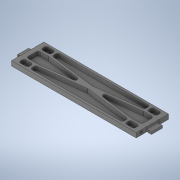
# Autodesk Inventor part: Cockpit_battery_front_frame
Saved by Autodesk Inventor 2020.4 (Build 244396000, 396)
## iProperties
Created: 2022-01-28
Part Number: Cockpit_battery_front_frame
Material: アセタール樹脂、黒
Document SubType Name: Modeling
Designer: Masato Kubotera
Density: 1.425 g/cm^3
Appearance: 滑らか - 黒
Description: POM T5
Author: Masato Kubotera
Autodesk Inventor part; units mm, degrees
ref_plane "XZ Plane" through (0, 0, 0) normal (0, 1, 0) x (-1, 0, 0)
ref_plane "XY Plane" through (0, 0, 0) normal (0, 0, 1) x (1, 0, 0)
derived "Cockpit_side_frame.ipt"
sketch "スケッチ2" plane through (0, 0, 0) normal (0, 1, 0) x (-1, 0, 0)
  line L0 (-28.5, -22.5) -> (86.5, -22.5) construction
  line L1 (86.5, -22.5) -> (86.5, -138.5)
  line L2 (86.5, -96) -> (-28.5, -96) construction
  line L3 (-28.5, -96) -> (-28.5, -22.5) construction
  line L4 (-28.5, -22.5) -> (86.5, -96) construction
  line L5 (86.5, -22.5) -> (-28.5, -96) construction
  line L6 (36.5, -101) -> (36.5, -133.5)
  line L7 (41.5, -138.5) -> (86.5, -138.5)
  arc A0 (62.6349, -67.15) -> (61.15, -68.6349) centre (61.8925, -67.8925) ccw
  arc A1 (71.15, -69.2849) -> (69.6651, -67.8) centre (70.4075, -68.5425) ccw
  line L8 (63.3349, -67.8) -> (69.6651, -67.8)
  line L9 (62.6349, -67.15) -> (70.3651, -67.15)
  line L10 (61.9, -67.85) -> (71.1, -67.85) construction
  arc A2 (63.3349, -67.8) -> (61.85, -69.2849) centre (62.5925, -68.5425) ccw
  line L11 (61.2, -67.2) -> (71.8, -67.2) construction
  line L12 (71.15, -69.2849) -> (71.15, -80.2151)
  line L13 (71.8, -74.75) -> (61.2, -74.75) construction
  line L14 (71.85, -68.6349) -> (71.85, -80.8651)
  line L15 (71.1, -67.85) -> (71.1, -81.65) construction
  line L16 (61.85, -69.2849) -> (61.85, -80.2151)
  line L17 (71.8, -67.2) -> (71.8, -82.3) construction
  line L18 (61.15, -68.6349) -> (61.15, -80.8651)
  line L19 (66.5, -67.2) -> (66.5, -82.3) construction
  line L20 (61.9, -81.65) -> (61.9, -67.85) construction
  line L21 (71.1, -67.85) -> (61.9, -81.65) construction
  line L22 (71.8, -67.2) -> (61.2, -82.3) construction
  line L23 (61.2, -67.2) -> (71.8, -82.3) construction
  line L24 (61.2, -82.3) -> (61.2, -67.2) construction
  line L25 (61.9, -67.85) -> (71.1, -81.65) construction
  arc A3 (71.85, -68.6349) -> (70.3651, -67.15) centre (71.1075, -67.8925) ccw
  line L26 (71.1, -81.65) -> (61.9, -81.65) construction
  line L27 (71.8, -82.3) -> (61.2, -82.3) construction
  arc A4 (61.85, -80.2151) -> (63.3349, -81.7) centre (62.5925, -80.9575) ccw
  arc A5 (61.15, -80.8651) -> (62.6349, -82.35) centre (61.8925, -81.6075) ccw
  line L28 (63.3349, -81.7) -> (69.6651, -81.7)
  line L29 (62.6349, -82.35) -> (70.3651, -82.35)
  arc A6 (69.6651, -81.7) -> (71.15, -80.2151) centre (70.4075, -80.9575) ccw
  arc A7 (70.3651, -82.35) -> (71.85, -80.8651) centre (71.1075, -81.6075) ccw
  line L30 (-23.5, -22.5) -> (-28.5, -27.5)
  line L31 (-28.5, -59.25) -> (86.5, -59.25) construction
  line L32 (29, -22.5) -> (29, -96) construction
  line L33 (-23.5, -96) -> (-28.5, -91)
  line L34 (-28.5, -27.5) -> (-28.5, -91)
  line L35 (-21, -25) -> (-26, -25) construction
  line L36 (-26, -25) -> (-26, -93.5) construction
  line L37 (-26, -93.5) -> (-21, -93.5) construction
  line L38 (-21, -93.5) -> (-21, -25) construction
  line L39 (-21, -25) -> (-26, -93.5) construction
  line L40 (-26, -25) -> (-21, -93.5) construction
  line L41 (-26.05, -46.7) -> (-20.95, -46.7)
  line L42 (-20.95, -46.7) -> (-20.95, -71.8)
  line L43 (-20.95, -71.8) -> (-26.05, -71.8)
  line L44 (-26.05, -71.8) -> (-26.05, -46.7)
  line L45 (-26.05, -46.7) -> (-20.95, -71.8) construction
  line L46 (-20.95, -46.7) -> (-26.05, -71.8) construction
  line L47 (-26, -46.75) -> (-21, -46.75) construction
  line L48 (-26, -71.75) -> (-21, -71.75) construction
  line L49 (-23.5, -25) -> (-23.5, -93.5) construction
  circle A8 centre (-23.5, -35) radius 3
  circle A9 centre (-23.5, -35) radius 1.6
  arc A10 (-24.5651, -46.7) -> (-26.05, -48.1849) centre (-25.3075, -47.4425) ccw
  arc A11 (-20.95, -48.1849) -> (-22.4349, -46.7) centre (-21.6925, -47.4425) ccw
  arc A12 (-22.4349, -71.8) -> (-20.95, -70.3151) centre (-21.6925, -71.0575) ccw
  arc A13 (-26.05, -70.3151) -> (-24.5651, -71.8) centre (-25.3075, -71.0575) ccw
  circle A14 centre (-23.5, -83.5) radius 1.6
  circle A15 centre (-23.5, -83.5) radius 3
  line L50 (31.5, -96) -> (36.5, -101)
  line L51 (-23.5, -96) -> (31.5, -96)
  line L52 (79, -61) -> (-21, -61) construction
  line L53 (-21, -61) -> (-21, -56) construction
  line L54 (-21, -56) -> (79, -56) construction
  line L55 (79, -56) -> (79, -61) construction
  line L56 (79, -61) -> (-21, -56) construction
  line L57 (-21, -61) -> (79, -56) construction
  line L58 (-21, -58.5) -> (79, -58.5) construction
  line L59 (29, -56) -> (29, -61) construction
  line L60 (4, -56) -> (4, -61) construction
  line L61 (54.05, -55.95) -> (3.95, -55.95)
  line L62 (3.95, -55.95) -> (3.95, -61.05)
  line L63 (3.95, -61.05) -> (54.05, -61.05)
  line L64 (54.05, -61.05) -> (54.05, -55.95)
  line L65 (54.05, -55.95) -> (3.95, -61.05) construction
  line L66 (3.95, -55.95) -> (54.05, -61.05) construction
  arc A16 (5.4349, -55.95) -> (3.95, -57.4349) centre (4.6925, -56.6925) ccw
  circle A17 centre (-3.5, -58.5) radius 3
  circle A18 centre (-3.5, -58.5) radius 1.6
  line L67 (54, -56) -> (54, -61) construction
  arc A19 (54.05, -57.4349) -> (52.5651, -55.95) centre (53.3075, -56.6925) ccw
  circle A20 centre (61.5, -58.5) radius 3
  circle A21 centre (61.5, -58.5) radius 1.6
  arc A22 (3.95, -59.5651) -> (5.4349, -61.05) centre (4.6925, -60.3075) ccw
  arc A23 (52.5651, -61.05) -> (54.05, -59.5651) centre (53.3075, -60.3075) ccw
  line L68 (-21, -88.5) -> (79, -88.5) construction
  line L69 (79, -88.5) -> (79, -93.5) construction
  line L70 (79, -93.5) -> (-21, -93.5) construction
  line L71 (-21, -93.5) -> (-21, -88.5) construction
  line L72 (-21, -88.5) -> (79, -93.5) construction
  line L73 (79, -88.5) -> (-21, -93.5) construction
  line L74 (-21, -91) -> (79, -91) construction
  line L75 (29, -88.5) -> (29, -93.5) construction
  line L76 (54.05, -91.05) -> (3.95, -91.05)
  line L77 (3.95, -91.05) -> (3.95, -88.45)
  line L78 (3.95, -88.45) -> (54.05, -88.45)
  line L79 (54.05, -88.45) -> (54.05, -91.05)
  line L80 (54.05, -91.05) -> (3.95, -88.45) construction
  line L81 (3.95, -91.05) -> (54.05, -88.45) construction
  line L82 (4, -88.5) -> (4, -91) construction
  line L83 (54, -88.5) -> (54, -91) construction
  line L84 (4, -89.75) -> (54, -89.75) construction
  arc A24 (6.05, -88.45) -> (3.95, -88.45) centre (5, -88.45) ccw
  arc A25 (54.05, -88.45) -> (51.95, -88.45) centre (53, -88.45) ccw
  arc A26 (51.95, -91.05) -> (54.05, -91.05) centre (53, -91.05) ccw
  arc A27 (3.95, -91.05) -> (6.05, -91.05) centre (5, -91.05) ccw
  circle A28 centre (-3.5, -91) radius 3
  circle A29 centre (-3.5, -91) radius 1.6
  circle A30 centre (61.5, -91) radius 3 construction
  circle A31 centre (61.5, -91) radius 1.6 construction
  line L85 (-23.5, -22.5) -> (64.25, -22.5)
  line L86 (64.25, -22.5) -> (64.25, -17.5)
  line L87 (64.25, -17.5) -> (72.25, -17.5)
  line L88 (72.25, -17.5) -> (72.25, -22.5)
  line L89 (72.25, -22.5) -> (79, -22.5)
  line L90 (79, -22.5) -> (79, -17.5)
  line L91 (86.5, -22.5) -> (86.5, -20)
  line L92 (79, -17.5) -> (84, -17.5)
  line L93 (84, -17.5) -> (86.5, -20)
  line L94 (68.25, -17.5) -> (68.25, -22.5) construction
  arc A32 (62.7651, -22.5) -> (64.25, -21.0151) centre (63.5075, -21.7575) ccw
  arc A33 (72.25, -21.0151) -> (73.7349, -22.5) centre (72.9925, -21.7575) ccw
  arc A34 (77.5151, -22.5) -> (79, -21.0151) centre (78.2575, -21.7575) ccw
  line L95 (-16, -88.5) -> (-16, -68.5) construction
  line L96 (-16, -68.5) -> (64, -68.5) construction
  line L97 (64, -68.5) -> (64, -88.5) construction
  line L98 (45.5, -86) -> (-16.5, -86)
  line L99 (-18.5, -84) -> (-18.5, -65.5)
  line L100 (-16.5, -63.5) -> (45.5, -63.5)
  line L101 (47.5, -65.5) -> (47.5, -84)
  line L102 (47.5, -86) -> (-18.5, -63.5) construction
  line L103 (-18.5, -86) -> (47.5, -63.5) construction
  arc A35 (-16.5, -63.5) -> (-18.5, -65.5) centre (-16.5, -65.5) ccw
  arc A36 (-18.5, -84) -> (-16.5, -86) centre (-16.5, -84) ccw
  arc A37 (45.5, -86) -> (47.5, -84) centre (45.5, -84) ccw
  arc A38 (47.5, -65.5) -> (45.5, -63.5) centre (45.5, -65.5) ccw
  line L104 (36.5, -133.5) -> (41.5, -138.5)
  line L105 (44, -131) -> (39, -131) construction
  line L106 (39, -131) -> (39, -96) construction
  line L107 (39, -96) -> (44, -96) construction
  line L108 (44, -96) -> (44, -131) construction
  line L109 (44, -131) -> (39, -96) construction
  line L110 (39, -131) -> (44, -96) construction
  line L111 (41.5, -96) -> (41.5, -131) construction
  line L112 (39, -113.5) -> (44, -113.5) construction
  line L113 (41.5, -107.5) -> (44, -107.5) construction
  line L114 (41.45, -107.45) -> (44.05, -107.45)
  line L115 (44.05, -107.45) -> (44.05, -119.55)
  line L116 (44.05, -119.55) -> (41.45, -119.55)
  line L117 (41.45, -119.55) -> (41.45, -107.45)
  line L118 (41.45, -107.45) -> (44.05, -119.55) construction
  line L119 (44.05, -107.45) -> (41.45, -119.55) construction
  arc A39 (44.05, -109.55) -> (44.05, -107.45) centre (44.05, -108.5) ccw
  arc A40 (42.9349, -107.45) -> (41.45, -108.9349) centre (42.1925, -108.1925) ccw
  arc A41 (44.05, -119.55) -> (44.05, -117.45) centre (44.05, -118.5) ccw
  line L120 (41.5, -119.5) -> (44, -119.5) construction
  arc A42 (41.45, -118.0651) -> (42.9349, -119.55) centre (42.1925, -118.8075) ccw
  line L121 (42.75, -107.5) -> (42.75, -119.5) construction
  circle A43 centre (41.5, -125.5) radius 3 construction
  circle A44 centre (41.5, -125.5) radius 1.6 construction
  circle A45 centre (41.5, -101.5) radius 3
  circle A46 centre (41.5, -101.5) radius 1.6
  circle A47 centre (-13.5, -55) radius 2
  line L122 (39, -131) -> (77.8645, -131) construction
  line L123 (77.8645, -131) -> (77.8645, -136) construction
  line L124 (77.8645, -136) -> (39, -136) construction
  line L125 (39, -136) -> (39, -131) construction
  line L126 (39, -131) -> (77.8645, -136) construction
  line L127 (77.8645, -131) -> (39, -136) construction
  line L128 (39, -133.5) -> (77.8645, -133.5) construction
  line L129 (58.4322, -131) -> (58.4322, -136) construction
  line L130 (58.4322, -133.5) -> (58.4322, -131) construction
  line L131 (50.8822, -130.95) -> (65.9822, -130.95)
  line L132 (65.9822, -130.95) -> (65.9822, -133.55)
  line L133 (65.9822, -133.55) -> (50.8822, -133.55)
  line L134 (50.8822, -133.55) -> (50.8822, -130.95)
  line L135 (50.8822, -130.95) -> (65.9822, -133.55) construction
  line L136 (65.9822, -130.95) -> (50.8822, -133.55) construction
  line L137 (50.9322, -131) -> (50.9322, -133.5) construction
  arc A48 (52.9822, -130.95) -> (50.8822, -130.95) centre (51.9322, -130.95) ccw
  arc A49 (50.8822, -132.0651) -> (52.3672, -133.55) centre (51.6247, -132.8075) ccw
  arc A50 (65.9822, -130.95) -> (63.8822, -130.95) centre (64.9322, -130.95) ccw
  arc A51 (64.4973, -133.55) -> (65.9822, -132.0651) centre (65.2398, -132.8075) ccw
  line L138 (65.9322, -131) -> (65.9322, -133.5) construction
  line L139 (50.9322, -132.25) -> (65.9322, -132.25) construction
  circle A52 centre (72.4322, -133.5) radius 1.6 construction
  circle A53 centre (72.4322, -133.5) radius 3 construction
  circle A54 centre (44.4322, -133.5) radius 3
  circle A55 centre (44.4322, -133.5) radius 1.6
  line L140 (48.5, -96) -> (77, -96)
  line L141 (79, -98) -> (79, -126.5)
  line L142 (77, -128.5) -> (48.5, -128.5)
  line L143 (46.5, -126.5) -> (46.5, -98)
  line L144 (46.5, -96) -> (79, -128.5) construction
  line L145 (79, -96) -> (46.5, -128.5) construction
  arc A56 (48.5, -96) -> (46.5, -98) centre (48.5, -98) ccw
  arc A57 (46.5, -126.5) -> (48.5, -128.5) centre (48.5, -126.5) ccw
  arc A58 (77, -128.5) -> (79, -126.5) centre (77, -126.5) ccw
  arc A59 (79, -98) -> (77, -96) centre (77, -98) ccw
  line L146 (79, -91.1738) -> (84, -91.1738) construction
  line L147 (84, -91.1738) -> (84, -136) construction
  line L148 (84, -136) -> (79, -136) construction
  line L149 (79, -136) -> (79, -91.1738) construction
  line L150 (79, -91.1738) -> (84, -136) construction
  line L151 (84, -91.1738) -> (79, -136) construction
  line L152 (81.5, -91.1738) -> (81.5, -136) construction
  circle A60 centre (81.5, -93.6738) radius 1.475
  circle A61 centre (81.5, -98.6738) radius 1.475
  circle A62 centre (81.5, -103.6738) radius 1.475
  circle A63 centre (81.5, -133.5) radius 1.6
  arc A64 (84, -91.1738) -> (79, -91.1738) centre (81.5, -133.5) ccw construction
  arc A65 (84.0111, -91.0742) -> (78.9889, -91.0742) centre (81.5, -133.5) ccw construction
  line L153 (86.5, -133.5) -> (81.5, -138.5)
  arc A66 (79, -131) -> (84, -136) centre (81.5, -133.5) ccw construction
  line L154 (79, -58.5) -> (84, -58.5) construction
  line L155 (84, -58.5) -> (84, -91) construction
  line L156 (84, -91) -> (79, -91) construction
  line L157 (79, -91) -> (79, -58.5) construction
  line L158 (79, -58.5) -> (84, -91) construction
  line L159 (84, -58.5) -> (79, -91) construction
  line L160 (79, -74.75) -> (84, -74.75) construction
  line L161 (81.5, -58.5) -> (81.5, -91) construction
  line L162 (79, -69.75) -> (84, -69.75) construction
  line L163 (78.95, -69.7) -> (86.5, -69.7)
  line L164 (84.05, -69.7) -> (84.05, -79.8) construction
  line L165 (84.05, -79.8) -> (78.95, -79.8)
  line L166 (78.95, -79.8) -> (78.95, -69.7)
  line L167 (78.95, -69.7) -> (84.05, -79.8) construction
  line L168 (84.05, -69.7) -> (78.95, -79.8) construction
  arc A67 (80.4349, -69.7) -> (78.95, -71.1849) centre (79.6925, -70.4425) ccw
  arc A68 (78.95, -78.3151) -> (80.4349, -79.8) centre (79.6925, -79.0575) ccw
  line L169 (79, -79.75) -> (84, -79.75) construction
  circle A69 centre (81.5, -64.75) radius 1.6
  circle A70 centre (81.5, -64.75) radius 3
  circle A71 centre (81.5, -84.75) radius 1.6
  circle A72 centre (81.5, -84.75) radius 3
  line L170 (84.05, -79.8) -> (86.5, -79.8)
  circle A73 centre (81.5, -133.5) radius 3
  line L171 (75.625, -22.5) -> (75.625, -27.147) construction
  line L172 (60.875, -22.5) -> (60.875, -27.147) construction
  line L173 (64.25, -22.5) -> (72.25, -22.5)
  line L174 (-13.5, -29.5) -> (-13.5, -49)
  line L175 (-11.5, -51) -> (45.5, -51)
  line L176 (47.5, -49) -> (47.5, -29.5)
  line L177 (45.5, -27.5) -> (-11.5, -27.5)
  arc A74 (-11.5, -27.5) -> (-13.5, -29.5) centre (-11.5, -29.5) ccw
  arc A75 (-13.5, -49) -> (-11.5, -51) centre (-11.5, -49) ccw
  arc A76 (45.5, -51) -> (47.5, -49) centre (45.5, -49) ccw
  arc A77 (47.5, -29.5) -> (45.5, -27.5) centre (45.5, -29.5) ccw
  point P0 (0, 0)
  point P1 (29, -59.25)
  point P2 (-25.7227, -96)
  point P3 (61.85, -67.8)
  point P4 (61.15, -67.15)
  point P5 (66.5, -74.75)
  point P6 (-23.5, -59.25)
  point P7 (29, -58.5)
  point P8 (29, -91)
  point P9 (29, -89.75)
  point P10 (29, -89.75)
  point P11 (52.5, -22)
  point P12 (14.5, -74.75)
  point P13 (-18.5, -61)
  point P14 (47.5, -61)
  point P15 (41.5, -113.5)
  point P16 (42.75, -113.5)
  point P17 (58.4322, -133.5)
  point P18 (58.4322, -132.25)
  point P19 (62.75, -112.25)
  point P20 (81.5, -113.5869)
  point P21 (81.5, -74.75)
  point P22 (-13.5, -51)
  point P23 (47.5, -27.5)
  point P24 (-13.5, -27.5)
  dimension "d1" = 44
  dimension "d2" = 5
  dimension "d3" = 2.5
  measures "d1" horizontal distance of L107.end point (0, 0)
  measures "d2" distance of L107.end L106.end
  measures "d3" distance of L113.start L113.end
ref_plane "作業平面1" through (-44, 0, 0) normal (1, 0, 0) x (0, 1, 0)
sketch "スケッチ3" plane through (-44, 0, 0) normal (1, 0, 0) x (0, 1, 0)
  line L0 (-135, -131) -> (0, -131)
  line L1 (0, -131) -> (0, -96)
  line L2 (0, -96) -> (-135, -96)
  line L3 (-135, -96) -> (-135, -131)
  line L4 (-135, -131) -> (0, -96) construction
  line L5 (0, -131) -> (-135, -96) construction
  line L6 (0, -107.5) -> (5, -107.5)
  line L7 (5, -107.5) -> (5, -119.5)
  line L8 (5, -119.5) -> (0, -119.5)
  line L9 (0, -113.5) -> (-135, -113.5) construction
  line L10 (-67.5, -96) -> (-67.5, -131)
  arc A0 (0, -106.0151) -> (1.4849, -107.5) centre (0.7425, -106.7575) ccw
  line L11 (-7, -98.5) -> (-13, -98.5)
  line L12 (-15, -100.5) -> (-15, -102.5)
  line L13 (-13, -104.5) -> (-7, -104.5)
  line L14 (-5, -102.5) -> (-5, -100.5)
  line L15 (-5, -98.5) -> (-15, -104.5) construction
  line L16 (-15, -98.5) -> (-5, -104.5) construction
  line L17 (-17.5, -100.5) -> (-17.5, -102.8772)
  line L18 (-16.1233, -107) -> (-7, -107)
  line L19 (-5, -109) -> (-5, -118)
  line L20 (-16.3757, -107.016) -> (-51.7468, -111.516)
  line L21 (-67.2476, -110.9679) -> (-19.2476, -104.8612)
  line L22 (-19.5, -98.5) -> (-67.5, -98.5)
  line L23 (-5, -101.5) -> (0, -101.5) construction
  line L24 (-7, -128.5) -> (-13, -128.5)
  line L25 (-15, -126.5) -> (-15, -124.5)
  line L26 (-13, -122.5) -> (-7, -122.5)
  line L27 (-5, -124.5) -> (-5, -126.5)
  line L28 (-17.5, -126.5) -> (-17.5, -124.1228)
  line L29 (-16.1233, -120) -> (-7, -120)
  line L30 (-16.3757, -119.984) -> (-51.7468, -115.484)
  line L31 (-67.2476, -116.0321) -> (-19.2476, -122.1388)
  line L32 (-19.5, -128.5) -> (-67.5, -128.5)
  line L33 (-128, -98.5) -> (-122, -98.5)
  line L34 (-120, -100.5) -> (-120, -102.5)
  line L35 (-122, -104.5) -> (-128, -104.5)
  line L36 (-130, -102.5) -> (-130, -100.5)
  line L37 (-117.5, -100.5) -> (-117.5, -102.8772)
  line L38 (-118.8767, -107) -> (-128, -107)
  line L39 (-130, -109) -> (-130, -118)
  line L40 (-118.6243, -107.016) -> (-83.2532, -111.516)
  line L41 (-67.7524, -110.9679) -> (-115.7524, -104.8612)
  line L42 (-115.5, -98.5) -> (-67.5, -98.5)
  line L43 (-128, -128.5) -> (-122, -128.5)
  line L44 (-130, -124.5) -> (-130, -126.5)
  line L45 (-122, -122.5) -> (-128, -122.5)
  line L46 (-120, -126.5) -> (-120, -124.5)
  line L47 (-117.5, -126.5) -> (-117.5, -124.1228)
  line L48 (-115.5, -128.5) -> (-67.5, -128.5)
  line L49 (-67.7524, -116.0321) -> (-115.7524, -122.1388)
  line L50 (-118.6243, -119.984) -> (-83.2532, -115.484)
  line L51 (-118.8767, -120) -> (-128, -120)
  arc A1 (-5, -100.5) -> (-7, -98.5) centre (-7, -100.5) ccw
  arc A2 (-13, -98.5) -> (-15, -100.5) centre (-13, -100.5) ccw
  arc A3 (-15, -102.5) -> (-13, -104.5) centre (-13, -102.5) ccw
  arc A4 (-7, -104.5) -> (-5, -102.5) centre (-7, -102.5) ccw
  arc A5 (-19.2476, -104.8612) -> (-17.5, -102.8772) centre (-19.5, -102.8772) ccw
  arc A6 (-17.5, -100.5) -> (-19.5, -98.5) centre (-19.5, -100.5) ccw
  arc A7 (-115.5, -98.5) -> (-117.5, -100.5) centre (-115.5, -100.5) ccw
  arc A8 (-117.5, -102.8772) -> (-115.7524, -104.8612) centre (-115.5, -102.8772) ccw
  arc A9 (-67.7524, -110.9679) -> (-67.2476, -110.9679) centre (-67.5, -108.9839) ccw
  arc A10 (-51.7468, -111.516) -> (-51.7468, -115.484) centre (-51.4944, -113.5) ccw
  arc A11 (-16.1233, -107) -> (-16.3757, -107.016) centre (-16.1233, -109) ccw
  arc A12 (-5, -109) -> (-7, -107) centre (-7, -109) ccw
  arc A13 (-7, -120) -> (-5, -118) centre (-7, -118) ccw
  arc A14 (-16.3757, -119.984) -> (-16.1233, -120) centre (-16.1233, -118) ccw
  arc A15 (-13, -122.5) -> (-15, -124.5) centre (-13, -124.5) ccw
  arc A16 (-15, -126.5) -> (-13, -128.5) centre (-13, -126.5) ccw
  arc A17 (-7, -128.5) -> (-5, -126.5) centre (-7, -126.5) ccw
  arc A18 (-5, -124.5) -> (-7, -122.5) centre (-7, -124.5) ccw
  arc A19 (-19.5, -128.5) -> (-17.5, -126.5) centre (-19.5, -126.5) ccw
  arc A20 (-17.5, -124.1228) -> (-19.2476, -122.1388) centre (-19.5, -124.1228) ccw
  arc A21 (-67.2476, -116.0321) -> (-67.7524, -116.0321) centre (-67.5, -118.0161) ccw
  arc A22 (-122, -128.5) -> (-120, -126.5) centre (-122, -126.5) ccw
  arc A23 (-120, -124.5) -> (-122, -122.5) centre (-122, -124.5) ccw
  arc A24 (-128, -122.5) -> (-130, -124.5) centre (-128, -124.5) ccw
  arc A25 (-130, -126.5) -> (-128, -128.5) centre (-128, -126.5) ccw
  arc A26 (-117.5, -126.5) -> (-115.5, -128.5) centre (-115.5, -126.5) ccw
  arc A27 (-115.7524, -122.1388) -> (-117.5, -124.1228) centre (-115.5, -124.1228) ccw
  arc A28 (-130, -118) -> (-128, -120) centre (-128, -118) ccw
  arc A29 (-128, -107) -> (-130, -109) centre (-128, -109) ccw
  arc A30 (-118.6243, -107.016) -> (-118.8767, -107) centre (-118.8767, -109) ccw
  arc A31 (-83.2532, -115.484) -> (-83.2532, -111.516) centre (-83.5056, -113.5) ccw
  arc A32 (-130, -102.5) -> (-128, -104.5) centre (-128, -102.5) ccw
  arc A33 (-128, -98.5) -> (-130, -100.5) centre (-128, -100.5) ccw
  arc A34 (-120, -100.5) -> (-122, -98.5) centre (-122, -100.5) ccw
  arc A35 (-122, -104.5) -> (-120, -102.5) centre (-122, -102.5) ccw
  arc A36 (-118.8767, -120) -> (-118.6243, -119.984) centre (-118.8767, -118) ccw
  arc A37 (1.4849, -119.5) -> (0, -120.9849) centre (0.7425, -120.2425) ccw
  point P0 (0, 0)
  point P1 (-67.5, -113.5)
  point P2 (0, -107.5)
  point P3 (0, -107.5)
  point P4 (0, -107.5)
  point P5 (0, -119.5)
  point P6 (0, -119.5)
  point P7 (0, -119.5)
  point P8 (-10, -101.5)
  point P9 (-17.5, -98.5)
  point P10 (-16.25, -107)
  point P11 (-5, -107)
  point P12 (-67.3416, -113.5)
  point P13 (-67.5, -111)
  point P14 (-17.5, -104.6389)
  point P15 (-5, -128.5)
  point P16 (-15, -122.5)
  point P17 (-15, -128.5)
  point P18 (-5, -122.5)
  point P19 (-17.5, -128.5)
  point P20 (-16.25, -120)
  point P21 (-5, -120)
  point P22 (-67.5, -116)
  point P23 (-17.5, -122.3611)
  point P24 (-130, -98.5)
  point P25 (-120, -104.5)
  point P26 (-120, -98.5)
  point P27 (-130, -104.5)
  point P28 (-117.5, -98.5)
  point P29 (-118.75, -107)
  point P30 (-130, -107)
  point P31 (-67.6584, -113.5)
  point P32 (-117.5, -104.6389)
  point P33 (-130, -128.5)
  point P34 (-120, -128.5)
  point P35 (-130, -122.5)
  point P36 (-120, -122.5)
  point P37 (-117.5, -128.5)
  point P38 (-117.5, -122.3611)
  point P39 (-118.75, -120)
  point P40 (-130, -120)
  point P41 (-67.5, -110.9839)
  point P42 (-67.5, -116.0161)
  point P43 (0, -120.9849)
  point P44 (1.4849, -119.5)
  dimension "d5" = 1.05
  dimension "d6" = 5
  dimension "d7" = 135
  dimension "d8" = 2.5
  dimension "d9" = 2.5
  dimension "d10" = 5
  dimension "d11" = 2.5
  dimension "d14" = 5
  dimension "d15" = 2
  dimension "d16" = 10
  dimension "d17" = 2.5
  dimension "d18" = 11.25
  constraints: 104 end point, 79 point on line, 77 point on circle, 72 tangent, 38 centre point, 35 equal radius, 30 symmetric about line, 9 midpoint, 8 perpendicular, 5 parallel, 4 coincident, 3 horizontal, 2 collinear, 1 vertical, 1 other
  measures "d5" radius of A0
  measures "d6" distance of L6.start L6.end
  measures "d7" distance of L1.end L2.end
  measures "d8" vertical distance of L15.start L1.end
  measures "d9" distance of point (-5, -107) L16.end
  measures "d10" horizontal distance of L15.start L1.end
  measures "d11" distance of point (-17.5, -98.5) L16.start
  measures "d14" distance of point (-67.5, -116) point (-67.5, -111)
  measures "d15" radius of A1
  measures "d16" distance of L15.start L16.start
  measures "d17" distance between parallel lines of L21 L20
  measures "d18" distance of point (-5, -107) point (-16.25, -107)
extrude "押し出し1" add sketch "スケッチ3" along normal blind 5 contours L10 L32 A19 L28 A20 L31 A21 A9 L21 A5 L17 A6 L22 L2 L1 A0 A37 L0
extrude "押し出し2" add sketch "スケッチ3" along normal blind 2.5 contours L1 A0 L6 L7 L8 A37
extrude "押し出し3" add sketch "スケッチ3" along normal blind 0.5 contours L10 A21 L31 A20 L28 A19 L32 | L22 A6 L17 A5 L21 A9 L10 | A1 L14 A4 L13 A3 L12 A2 L11 | L18 A12 L19 A13 L29 A14 L30 A10 L20 A11 | L24 A16 L25 A15 L26 A18 L27 A17
hole "穴1" at (-41.5, 0, -101.5) direction (0, -1, 0) diameter 3.4587 depth 5 thread size "M4x0.5" class "6H" standard "ISO Metric profile"
mirror "ミラー1" about plane through (-44, -67.5, -128.5) normal (0, -1, 0)
equation "\"d9\" = d8"
equation "\"d11\" = d8"
equation "\"d18\" = d16 + 0.5 * d11"
equation "\"d19\" = d2"
equation "\"d21\" = d3"
equation "\"d4\" = -d1"
